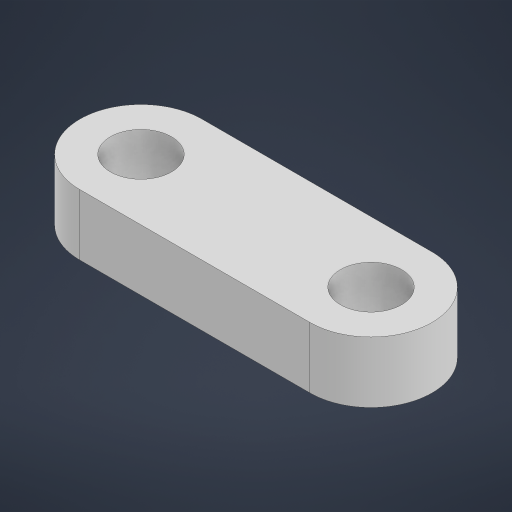
# Autodesk Inventor part: link
Saved by Autodesk Inventor 2024.3 (Build 283343000, 343)
## iProperties
Created: 2024-09-28
Part Number: link
Material: Generic
Document SubType Name: Modeling
Designer: sam
Density: 1 g/cm^3
Appearance: Default
Author: sam
Autodesk Inventor part; units mm, degrees
ref_plane "YZ Plane" through (0, 0, 0) normal (1, 0, 0) x (0, 1, 0)
ref_plane "XZ Plane" through (0, 0, 0) normal (0, 1, 0) x (-1, 0, 0)
ref_plane "XY Plane" through (0, 0, 0) normal (0, 0, 1) x (1, 0, 0)
sketch "Sketch1" plane through (0, 0, 0) normal (0, 1, 0) x (-1, 0, 0)
  line L0 (-9.422, -5) -> (9.422, -5)
  line L1 (14.422, 0) -> (14.422, 0)
  line L2 (9.422, 5) -> (-9.422, 5)
  line L3 (-14.422, 0) -> (-14.422, 0)
  line L4 (-14.422, -5) -> (14.422, 5) construction
  line L5 (14.422, -5) -> (-14.422, 5) construction
  circle A0 centre (9.422, 0) radius 2.5
  circle A1 centre (-9.422, 0) radius 2.5
  arc A2 (9.422, -5) -> (14.422, 0) centre (9.422, 0) ccw
  arc A3 (14.422, 0) -> (9.422, 5) centre (9.422, 0) ccw
  arc A4 (-9.422, 5) -> (-14.422, 0) centre (-9.422, 0) ccw
  arc A5 (-14.422, 0) -> (-9.422, -5) centre (-9.422, 0) ccw
  point P0 (0, 0)
  point P1 (14.422, 0)
  point P2 (-14.422, 0)
  dimension "d0" = 10
  dimension "d1" = 28.844
  dimension "d3" = 5
  dimension "d4" = 5
  dimension "d5" = 5
  dimension "d6" = 5
  dimension "d7" = 5
  dimension "d8" = 5
  dimension "d9" = 5
  constraints: 12 end point, 8 point on circle, 8 point on line, 8 tangent, 6 centre point, 3 equal radius, 2 midpoint, 2 parallel, 1 horizontal, 1 perpendicular
  measures "d0" distance of L4.end L5.start
  measures "d1" distance between parallel lines of L3 L1
  measures "d3" diameter of A0
  measures "d4" diameter of A1
  measures "d5" distance from line of L3 A1.centre
  measures "d6" distance from line of L1 A0.centre
  measures "d7" distance from line of L2 A1.centre
  measures "d8" distance from line of L2 A0.centre
  measures "d9" radius of A2
extrude "Extrusion1" add sketch "Sketch1" along normal blind 5
body "Solid1"
